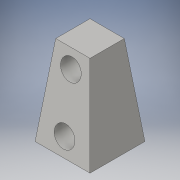
# Autodesk Inventor part: twoHoleWriteSupport
Saved by Autodesk Inventor 2016 SP1 (Build 200210100, 210)
## iProperties
Created: 2015-12-14
Part Number: twoHoleWriteSupport
Material: Generic
Document SubType Name: Modeling
Designer: steele
Density: 1 g/cm^3
Appearance: Default
Author: steele
Autodesk Inventor part; units mm, degrees
ref_plane "YZ Plane" through (0, 0, 0) normal (1, 0, 0) x (0, 1, 0)
sketch "Sketch2" plane through (0, 0, 0) normal (0, 1, 0) x (-1, 0, 0)
  line L0 (-12.7, 12.7) -> (-12.7, -12.7)
  line L1 (-12.7, -12.7) -> (12.7, -12.7)
  line L2 (12.7, -12.7) -> (12.7, 12.7)
  line L3 (12.7, 12.7) -> (-12.7, 12.7)
  line L4 (-12.7, 12.7) -> (12.7, -12.7) construction
  line L5 (-12.7, -12.7) -> (12.7, 12.7) construction
  point P0 (0, 0)
  dimension "d2" = 25.4
  dimension "d3" = 25.4
  constraints: 12 end point, 2 midpoint, 2 parallel, 1 perpendicular, 1 vertical
  measures "d2" distance of L0.end L1.end
  measures "d3" distance of L1.end L2.end
ref_plane "Work Plane1" through (0, 41.275, 0) normal (0, 1, 0) x (-1, 0, 0)
sketch "Sketch3" plane through (0, 41.275, 0) normal (0, 1, 0) x (-1, 0, 0)
  line L0 (-7.9375, 7.9375) -> (-7.9375, -7.9375)
  line L1 (-7.9375, -7.9375) -> (7.9375, -7.9375)
  line L2 (7.9375, -7.9375) -> (7.9375, 7.9375)
  line L3 (7.9375, 7.9375) -> (-7.9375, 7.9375)
  line L4 (-7.9375, 7.9375) -> (7.9375, -7.9375) construction
  line L5 (-7.9375, -7.9375) -> (7.9375, 7.9375) construction
  point P0 (0, 0)
  dimension "d5" = 15.875
  dimension "d6" = 15.875
  constraints: 12 end point, 2 midpoint, 2 parallel, 1 perpendicular, 1 vertical
  measures "d5" distance of L0.end L1.end
  measures "d6" distance of L1.end L2.end
loft "Loft1" add profiles "Sketch2", "Sketch3"
ref_plane "Work Plane2" through (12.7, 0, 12.7) normal (0, 0, 1) x (1, 0, 0)
sketch "Sketch5" plane through (12.7, 0, 12.7) normal (0, 0, 1) x (1, 0, 0)
  line L0 (-12.7, 0) -> (-12.7, 41.275) construction
  line L1 (-20.6375, 41.275) -> (-4.7625, 41.275) construction
  circle A0 centre (-12.7, 33.3375) radius 4.7625
  circle A1 centre (-12.7, 7.9375) radius 4.7625
  dimension "d17" = 9.525
  dimension "d19" = 7.9375
  dimension "d20" = 9.525
  dimension "d21" = 25.4
  constraints: 2 centre point, 2 end point, 2 point on line, 1 midpoint
  measures "d17" diameter of A0
  measures "d19" distance of L0.start A1.centre
  measures "d20" diameter of A1
  measures "d21" distance of A1.centre A0.centre
extrude "Extrusion2" cut sketch "Sketch5" against normal through all
equation "\"d2\" = baseWidth"
equation "\"d3\" = baseDepth"
equation "\"d5\" = baseForTopHoleWidth"
equation "\"d6\" = baseForTopHoleDepth"
equation "\"d17\" = topHoleDiam"
equation "\"d19\" = bottomHoleCenterHeight"
equation "\"d20\" = bottomHoleDiam"
equation "\"d21\" = deltaBetweenHoles"
equation "\"materialSupportWidth\" = 3.175"
equation "\"baseWidth\" = 25.4"
equation "\"baseDepth\" = 25.4"
equation "\"bottomHoleDiam\" = 9.525"
equation "\"bottomHoleRadius\" = 0.5 * bottomHoleDiam"
equation "\"washerDiam\" = 13.97"
equation "\"depthForSocketHead\" = 6.35"
equation "\"edgeToBoltHole\" = -0.5 * bottomHoleDiam + 0.5 * baseWidth"
equation "\"topHoleDiam\" = bottomHoleDiam"
equation "\"topHoleRadius\" = 0.5 * topHoleDiam"
equation "\"deltaBetweenHoles\" = 25.4"
equation "\"baseForTopHoleWidth\" = bottomHoleDiam + 2 * materialSupportWidth"
equation "\"baseForTopHoleDepth\" = bottomHoleDiam + 2 * materialSupportWidth"
equation "\"bottomHoleCenterHeight\" = 0.5 * bottomHoleDiam + materialSupportWidth"
equation "\"baseForTopHoleHeight\" = topHoleRadius + bottomHoleCenterHeight + deltaBetweenHoles + materialSupportWidth"
equation "\"topOfPyramid\" = topHoleDiam + baseForTopHoleHeight + 2 * materialSupportWidth"
equation "\"d4\" = baseForTopHoleHeight"
body "Solid1"
